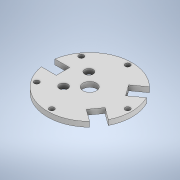
# Autodesk Inventor part: actuatorMountingPlate
Saved by Autodesk Inventor 2021 (Build 250183000, 183)
## iProperties
Created: 2021-01-06
Part Number: actuatorMountingPlate
Material: Generic
Document SubType Name: Modeling
Designer: awitc
Density: 1 g/cm^3
Appearance: Default
Author: awitc
Autodesk Inventor part; units mm, degrees
ref_plane "YZ Plane" through (0, 0, 0) normal (1, 0, 0) x (0, 1, 0)
ref_plane "XZ Plane" through (0, 0, 0) normal (0, 1, 0) x (-1, 0, 0)
ref_plane "XY Plane" through (0, 0, 0) normal (0, 0, 1) x (1, 0, 0)
sketch "Sketch1" plane through (0, 0, 0) normal (0, 1, 0) x (-1, 0, 0)
  line L0 (-17.6137, 17.7414) -> (-15.5618, 16.2506)
  line L1 (-23.5374, 22.0452) -> (-13.679, 22.0452) construction
  line L2 (-22.316, 11.2693) -> (-20.2641, 9.7784)
  line L3 (-22.316, -11.2693) -> (-20.2641, -9.7784)
  line L4 (-17.6137, -17.7414) -> (-15.5618, -16.2506)
  line L5 (24.6779, 4) -> (22.1416, 4)
  line L6 (24.6779, -4) -> (22.1416, -4)
  line L7 (-20.2641, -9.7784) -> (-19.2354, -9.0311)
  line L8 (-15.5618, -16.2506) -> (-14.5332, -15.5032)
  line L9 (-20.2641, 9.7784) -> (-19.2354, 9.0311)
  line L10 (-15.5618, 16.2506) -> (-14.5332, 15.5032)
  line L11 (22.1416, 4) -> (20.8701, 4)
  line L12 (22.1416, -4) -> (20.8701, -4)
  arc A0 (-17.6137, -17.7414) -> (24.6779, -4) centre (0, 0) ccw
  arc A1 (24.6779, 4) -> (-17.6137, 17.7414) centre (0, 0) ccw
  arc A2 (-22.316, 11.2693) -> (-22.316, -11.2693) centre (0, 0) ccw
  line L13 (20.8701, 4) -> (15.8701, 4)
  line L14 (15.8701, 4) -> (15.8701, -4)
  line L15 (15.8701, -4) -> (20.8701, -4)
  line L16 (-14.5332, 15.5032) -> (-10.4881, 12.5643)
  line L17 (-10.4881, 12.5643) -> (-15.1903, 6.0922)
  line L18 (-15.1903, 6.0922) -> (-19.2354, 9.0311)
  line L19 (-19.2354, -9.0311) -> (-15.1903, -6.0922)
  line L20 (-15.1903, -6.0922) -> (-10.4881, -12.5643)
  line L21 (-10.4881, -12.5643) -> (-14.5332, -15.5032)
  circle A3 centre (-22.5, 0) radius 1.5
  circle A4 centre (0, 22.5) radius 1.5
  circle A5 centre (18.2029, 13.2252) radius 1.5
  circle A6 centre (18.2029, -13.2252) radius 1.5
  circle A7 centre (0, -22.5) radius 1.5
  circle A8 centre (0, 0) radius 4
  line L22 (0, 0) -> (8, 0)
  line L23 (8, 0) -> (8, 7.5)
  line L24 (8, 0) -> (8, -7.5)
  circle A9 centre (8, -7.5) radius 2.5
  circle A10 centre (8, 7.5) radius 2.5
  point P0 (-28.2397, -15.5731)
  point P1 (-23.5374, -22.0452)
  point P2 (32, -4)
  dimension "d1" = 36
  dimension "d3" = 5
  dimension "d4" = 5
  dimension "d6" = 3
  dimension "d7" = 3
  dimension "d8" = 3
  dimension "d9" = 3
  dimension "d10" = 3
  dimension "d13" = 8
  dimension "d14" = 8
  dimension "d15" = 7.5
  dimension "d16" = 7.5
  dimension "d17" = 5
  dimension "d18" = 5
  constraints: 50 end point, 11 centre point, 6 point on circle, 5 parallel, 4 coincident, 4 horizontal, 4 perpendicular, 2 vertical
  measures "d1" angle of L0 L1
  measures "d3" distance of L15.end L14.end
  measures "d4" distance of L10.end L16.end
  measures "d6" diameter of A3
  measures "d7" diameter of A4
  measures "d8" diameter of A5
  measures "d9" diameter of A6
  measures "d10" diameter of A7
  measures "d13" diameter of A8
  measures "d14" distance of L22.start L22.end
  measures "d15" distance of L22.end L23.end
  measures "d16" distance of L22.end L24.end
  measures "d17" diameter of A9
  measures "d18" diameter of A10
extrude "Extrusion2" add sketch "Sketch1" along normal blind 3
body "Solid2"
